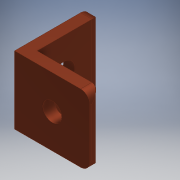
# Autodesk Inventor part: Cantoneira
Saved by Autodesk Inventor 2018 (Build 220112000, 112)
## iProperties
Created: 2018-07-06
Part Number: Cantoneira
Material: Cobre
Document SubType Name: Modeling
Designer: Regner
Density: 8.94 g/cm^3
Appearance: Cobre - Acetinado
Author: Regner
Autodesk Inventor part; units mm, degrees
ref_plane "YZ Plane" through (0, 0, 0) normal (1, 0, 0) x (0, 1, 0)
ref_plane "XZ Plane" through (0, 0, 0) normal (0, 1, 0) x (-1, 0, 0)
ref_plane "XY Plane" through (0, 0, 0) normal (0, 0, 1) x (1, 0, 0)
sketch "Esboço1" plane through (0, 0, 0) normal (0, 0, 1) x (1, 0, 0)
  line L0 (10, -10) -> (-10, -10)
  line L1 (-10, -10) -> (-10, 10)
  line L2 (-10, 10) -> (-7, 10)
  line L3 (10, -7) -> (10, -10)
  line L4 (10, -10) -> (-10, 10) construction
  line L5 (-10, -10) -> (10, 10) construction
  line L6 (10, -7) -> (-7, -7)
  line L7 (-7, 10) -> (-7, -7)
  line L8 (-7, -10) -> (-7, -10.3421)
  point P0 (0, 0)
  dimension "d0" = 20
  dimension "d1" = 20
  dimension "d4" = 3
  dimension "d8" = 45
  dimension "d9" = 17
  constraints: 18 end point, 3 perpendicular, 2 midpoint, 2 parallel, 2 point on line, 2 vertical, 1 horizontal
  measures "d0" distance of L1.end L5.end
  measures "d1" distance of L0.end L1.end
  measures "d4" distance between parallel lines of L0 L6
  measures "d8" angle of L3 L4
  measures "d9" distance between parallel lines of L8 L3
extrude "Extrusão1" add sketch "Esboço1" along normal mid plane 18
fillet "Arredondamento1" radius 2.5 6 edges at (-8.5, 10, 9) (-7, 10, 0) (-8.5, 10, -9) (10, -8.5, 9) (10, -7, 0) (10, -8.5, -9)
hole "Furo1" at (-7, 0, 0) direction (-1, 0, 0) diameter 6 end through all
hole "Furo2" at (0, -7, 0) direction (0, -1, 0) diameter 5 end through all
